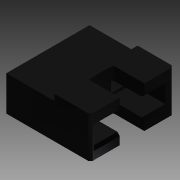
# Autodesk Inventor part: 68786-102LF
Saved by Autodesk Inventor 2013 (Build 170138000, 138)
## iProperties
Category: Control System
Company: Autodesk Inc.
Created: 2012-12-03
Part Number: 68786-102LF
Document SubType Name: Modeling
Designer: Autodesk Inc.
Density: 1 g/cm^3
Catalog Web Link: http://portal.fciconnect.com/portal/page/portal/FcicntPublic/ComergentConnect?appname=catDisplayStyle$domProductQueryName=68786-102lf*$OP=search
Vendor: FCI
Material: Generic
Description: Female, 2-pin shunt, black or white
Author: Autodesk Inc.
Autodesk Inventor part; units mm, degrees
ref_plane "YZ Plane" through (0, 0, 0) normal (1, 0, 0) x (0, 1, 0)
ref_plane "XZ Plane" through (0, 0, 0) normal (0, 1, 0) x (-1, 0, 0)
sketch "Sketch1" plane through (0, 0, 0) normal (0, 0, 1) x (1, 0, 0)
  line L0 (0, 0) -> (2.1082, 0)
  line L1 (2.1082, 0) -> (2.1082, 5.08)
  line L2 (2.1082, 5.08) -> (-0.381, 5.08)
  line L3 (-0.381, 5.08) -> (-0.381, 2.9029)
  line L4 (-0.381, 2.9029) -> (0, 2.9029)
  line L5 (0, 2.9029) -> (0, 0)
  dimension "d0" = 5.08
  dimension "d1" = 2.4892
  dimension "d2" = 2.1082
  dimension "d3" = 2.1771
  constraints: 12 end point, 4 parallel, 1 horizontal, 1 perpendicular
  measures "d0" distance of L0.end L1.end
  measures "d1" distance of L1.end L2.end
  measures "d2" distance of L0.start L0.end
  measures "d3" distance of L2.end L3.end
extrude "Extrusion1" add sketch "Sketch1" against normal blind 5.0292
sketch "Sketch2" plane through (0, 0, 0) normal (0, -1, 0) x (1, 0, 0)
  line L0 (0, -5.0292) -> (2.1082, -5.0292) projected
  line L1 (2.1082, 0) -> (2.1082, -5.0292) projected
  line L2 (0, 0) -> (2.1082, 0) projected
  line L3 (1.6742, -4.5242) -> (0.195, -4.5242)
  line L4 (0.195, -4.5242) -> (0.195, -3.045)
  line L5 (0.195, -3.045) -> (1.6742, -3.045)
  line L6 (1.6742, -3.045) -> (1.6742, -4.5242)
  line L7 (1.6742, -1.9842) -> (0.195, -1.9842)
  line L8 (0.195, -1.9842) -> (0.195, -0.505)
  line L9 (0.195, -0.505) -> (1.6742, -0.505)
  line L10 (1.6742, -0.505) -> (1.6742, -1.9842)
  line L11 (1.6742, -3.7846) -> (0.195, -3.7846) construction
  line L12 (0.195, -1.2446) -> (1.6742, -1.2446) construction
  line L13 (0.9346, -4.5242) -> (0.9346, -3.045) construction
  line L14 (0.5648, -3.4148) -> (0.5648, -4.1544)
  line L15 (0.5648, -4.1544) -> (1.3044, -4.1544)
  line L16 (1.3044, -4.1544) -> (1.3044, -3.4148)
  line L17 (1.3044, -3.4148) -> (0.5648, -3.4148)
  line L18 (0.5648, -0.8748) -> (0.5648, -1.6144)
  line L19 (0.5648, -1.6144) -> (1.3044, -1.6144)
  line L20 (1.3044, -1.6144) -> (1.3044, -0.8748)
  line L21 (1.3044, -0.8748) -> (0.5648, -0.8748)
  dimension "d6" = 1.4792
  dimension "d7" = 1.4792
  dimension "d8" = 1.2446
  dimension "d9" = 1.2446
  dimension "d10" = 1.4792
  dimension "d11" = 0.434
  dimension "d12" = 0.7396
  dimension "d13" = 0.7396
  constraints: 38 end point, 8 parallel, 6 midpoint, 4 perpendicular, 2 collinear, 2 horizontal, 6 other
  measures "d6" distance of L5.end L3.start
  measures "d7" distance of L9.end L7.start
  measures "d8" distance between parallel lines of L11 L0
  measures "d9" distance between parallel lines of L2 L12
  measures "d10" distance of L3.start L3.end
  measures "d11" distance between parallel lines of L6 L1
  measures "d12" distance of L15.end L16.end
  measures "d13" distance of L19.end L20.end
extrude "Extrusion2" cut sketch "Sketch2" against normal through all contours L17 L16 L15 L14 | L21 L20 L19 L18
chamfer "Chamfer1" distance 0.381 angle 45 8 edges at (0.5648, 0, -3.7846) (0.9346, 0, -3.4148) (1.3044, 0, -3.7846) (0.9346, 0, -4.1544) (0.9346, 0, -1.6144) (0.5648, 0, -1.2446) (0.9346, 0, -0.8748) (1.3044, 0, -1.2446)
sketch "Sketch3" plane through (-0.381, 5.08, 0) normal (0, 1, 0) x (1, 0, 0)
  line L0 (0.9458, 1.6144) -> (1.6854, 1.6144) projected
  line L1 (1.6854, 1.6144) -> (1.6854, 0.8748) projected
  line L2 (1.6854, 0.8748) -> (0.9458, 0.8748) projected
  line L3 (0.9458, 0.8748) -> (0.9458, 1.6144) projected
  line L4 (0.9458, 4.1544) -> (1.6854, 4.1544) projected
  line L5 (1.6854, 4.1544) -> (1.6854, 3.4148) projected
  line L6 (1.6854, 3.4148) -> (0.9458, 3.4148) projected
  line L7 (0.9458, 3.4148) -> (0.9458, 4.1544) projected
  line L8 (0, 0) -> (0, 5.0292) projected
  line L9 (2.4892, 0) -> (0, 0) projected
  line L10 (2.4892, 0) -> (2.4892, 5.0292) projected
  line L11 (1.8617, 0.3556) -> (1.8617, 4.6736)
  line L12 (1.8617, 4.6736) -> (0.7695, 4.6736)
  line L13 (0.7695, 4.6736) -> (0.7695, 0.3556)
  line L14 (0.7695, 0.3556) -> (1.8617, 0.3556)
  point P0 (0.381, 0)
  point P1 (0.7695, 2.5146)
  point P2 (0, 2.5146)
  point P3 (1.3156, 0.3556)
  point P4 (1.2446, 0)
  point P5 (1.3156, 0.8748)
  point P6 (0, 2.5146)
  dimension "d32" = 4.318
  dimension "d33" = 1.0922
  constraints: 8 end point, 6 midpoint, 3 parallel, 2 horizontal alignment, 1 horizontal, 1 vertical alignment
  measures "d32" distance of L11.start L11.end
  measures "d33" distance of L13.end L11.start
extrude "Extrusion3" cut sketch "Sketch3" against normal up to surface (2.1771 mm away)
sketch "Sketch4" plane through (-0.381, 2.9029, 0) normal (-1, 0, 0) x (0, 0, 1)
  line L0 (0, 2.1771) -> (-5.0292, 2.1771) projected
  line L1 (-3.2542, 2.1771) -> (-1.775, 2.1771)
  line L2 (-1.775, 2.1771) -> (-1.775, 0.2903)
  line L3 (-1.775, 0.2903) -> (-3.2542, 0.2903)
  line L4 (-3.2542, 0.2903) -> (-3.2542, 2.1771)
  point P0 (0, -2.9029)
  point P1 (-2.5146, 0.2903)
  point P2 (-2.5146, 2.1771)
  dimension "d24" = 1.4792
  dimension "d25" = 1.8869
  constraints: 8 end point, 2 midpoint, 2 parallel, 1 horizontal, 1 perpendicular, 1 point on line, 1 vertical alignment
  measures "d24" distance between parallel lines of L2 L4
  measures "d25" distance of L1.end L2.end
extrude "Extrusion4" cut sketch "Sketch4" against normal up to next
fillet "Fillet1" radius 0.127 2 edges at (0.0037, 3.1931, -1.775) (0.0037, 3.1931, -3.2542)
chamfer "Chamfer2" distance 0.127 angle 45 2 edges at (0.8636, 5.08, -5.0292) (0.8636, 5.08, 0)
ref_plane "Work Plane1" through (0.8636, 2.9029, -5.0292) normal (-1, 0, 0) x (0, 0, 1)
mirror "Mirror1" about plane through (0.8636, 2.9029, -5.0292) normal (-1, 0, 0) of "Extrusion4", "Fillet1"
chamfer "Chamfer3" distance 0.1524 angle 45 6 edges at (0.9346, 5.08, -0.3556) (0.3885, 5.08, -1.0653) (0.3885, 5.08, -3.9639) (0.9346, 5.08, -4.6736) (1.4807, 5.08, -3.9639) (1.4807, 5.08, -1.0653)
equation "\"d7\" = d6"
equation "\"d9\" = d8"
equation "\"d10\" = d6"
equation "\"d13\" = d12"
body "Solid1"
